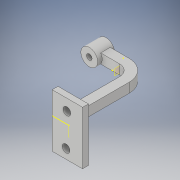
# Autodesk Inventor part: Base
Saved by Autodesk Inventor 2019 (Build 230136000, 136)
## iProperties
Created: 2019-05-09
Part Number: Base
Material: Generic
Document SubType Name: Modeling
Designer: riphipps21
Density: 1 g/cm^3
Appearance: Default
Author: riphipps21
Autodesk Inventor part; units mm, degrees
ref_plane "XZ Plane" through (0, 0, 0) normal (0, 1, 0) x (-1, 0, 0)
ref_plane "XY Plane" through (0, 0, 0) normal (0, 0, 1) x (1, 0, 0)
sketch "Sketch1" plane through (0, 0, 0) normal (0, 0, 1) x (1, 0, 0)
  point P0 (0, 0)
sketch "Sketch2" plane through (0, 0, 0) normal (0, 0, 1) x (1, 0, 0)
  circle A0 centre (-25.9578, 0) radius 5.461
  point P0 (0, 0)
  dimension "d30" = 10.922
  constraints: 1 centre point
  measures "d30" diameter of A0
extrude "Extrusion1" add sketch "Sketch2" along normal blind 12.7 and the other way blind 6.35
sketch "Sketch3" plane through (-25.9578, 0, 12.7) normal (0, 0, 1) x (1, 0, 0)
  point P0 (25.9578, 0)
  point P1 (0.0374, 0.0562)
hole "Hole1" at (-25.9204, 0.0562, 12.7) direction (0, 0, -1) diameter 6.2738 end through all
ref_plane "Work Plane1" through (3.175, 0, 0) normal (1, 0, 0) x (0, 1, 0)
sketch "Sketch4" plane through (3.175, 0, 0) normal (1, 0, 0) x (0, 1, 0)
  line L0 (5.461, -6.35) -> (5.461, 12.7) projected
  line L1 (5.461, 7.62) -> (-5.461, 7.62)
  line L2 (-5.461, 7.62) -> (-5.461, 4.445)
  line L3 (-5.461, 4.445) -> (5.461, 4.445)
  line L4 (5.461, 4.445) -> (5.461, 7.62)
  line L5 (5.461, 12.7) -> (-5.461, 12.7) projected
  line L6 (-5.461, -6.35) -> (-5.461, 12.7) projected
  point P0 (0, 0)
  dimension "d11" = 3.175
  dimension "d12" = 5.08
  constraints: 8 end point, 2 parallel, 1 collinear, 1 horizontal, 1 perpendicular, 1 point on line
  measures "d11" distance between parallel lines of L1 L3
  measures "d12" distance between parallel lines of L1 L5
sketch "Sketch5" plane through (0, 0, 0) normal (0, 1, 0) x (-1, 0, 0)
  line L0 (-3.175, -6.35) -> (-3.175, 12.7) projected
  arc A0 (-15.875, 20.32) -> (-3.175, 7.62) centre (-3.175, 20.32) ccw
  line L1 (-3.175, 20.32) -> (-15.875, 20.32) construction
  line L2 (31.4188, 12.7) -> (20.4968, 12.7) projected
  line L3 (-15.875, 20.32) -> (-15.875, 42.189)
  point P0 (0, 0)
  dimension "d13" = 12.7
  dimension "d14" = 5.08
  dimension "d15" = 0
  constraints: 4 end point, 2 point on circle, 1 centre point, 1 horizontal, 1 point on line, 1 vertical
  measures "d13" radius of A0
  measures "d14" distance from line of L2 A0.end
  measures "d15" distance from line of L1.start L0
sweep "Sweep1" add profiles "Sketch4" path "Sketch5" path curves A0 L3 contours L3 L2 L1 L0
sketch "Sketch8" plane through (3.175, 5.461, 7.62) normal (0, 1, 0) x (1, 0, 0)
  point P0 (-3.175, 7.62)
sketch "Sketch9" plane through (3.175, 5.461, 7.62) normal (0, 1, 0) x (1, 0, 0)
  point P0 (-3.175, 7.62)
sketch "Sketch10" plane through (3.175, 5.461, 7.62) normal (0, 1, 0) x (1, 0, 0)
  point P0 (-3.175, 7.62)
sketch "Sketch11" plane through (3.175, 5.461, 7.62) normal (0, 1, 0) x (1, 0, 0)
  point P0 (-3.175, 7.62)
sketch "Sketch12" plane through (3.175, 5.461, 7.62) normal (0, 1, 0) x (1, 0, 0)
  line L0 (12.7, -34.569) -> (15.875, -34.569) projected
  line L1 (12.7, -34.569) -> (15.875, -34.569)
  line L2 (15.875, -34.569) -> (15.875, -88.8996)
  line L3 (15.875, -88.8996) -> (12.7, -88.8996)
  line L4 (12.7, -88.8996) -> (12.7, -34.569)
  point P0 (-3.175, 7.62)
  constraints: 8 end point, 2 parallel, 1 horizontal, 1 perpendicular
sketch "Sketch13" plane through (3.175, 5.461, 7.62) normal (0, 1, 0) x (1, 0, 0)
  point P0 (-3.175, 7.62)
extrude "Extrusion4" add sketch "Sketch12" against normal blind 10.922
sketch "Sketch14" plane through (3.175, 5.461, 7.62) normal (0, 1, 0) x (1, 0, 0)
  line L0 (15.875, -88.8996) -> (12.7, -88.8996) projected
  line L1 (15.875, -88.8996) -> (31.877, -88.8996)
  line L2 (31.877, -88.8996) -> (31.877, -82.2956)
  line L3 (31.877, -82.2956) -> (15.875, -82.2956)
  line L4 (15.875, -82.2956) -> (15.875, -88.8996)
  point P0 (-3.175, 7.62)
  dimension "d36" = 6.604
  constraints: 8 end point, 2 parallel, 1 horizontal, 1 perpendicular
  measures "d36" distance of L1.end L2.end
extrude "Extrusion5" add sketch "Sketch14" against normal blind 10.922
sketch "Sketch15" plane through (3.175, 5.461, 7.62) normal (0, 1, 0) x (1, 0, 0)
  point P0 (-3.175, 7.62)
sketch "Sketch16" plane through (-25.9578, 0, 12.7) normal (0, 0, 1) x (1, 0, 0)
  point P0 (25.9578, 0)
sketch "Sketch17" plane through (-25.9578, 0, 12.7) normal (0, 0, 1) x (1, 0, 0)
  point P0 (25.9578, 0)
sketch "Sketch18" plane through (3.175, 5.461, 7.62) normal (0, 1, 0) x (1, 0, 0)
  point P0 (-3.175, 7.62)
sketch "Sketch19" plane through (3.175, 0, 0) normal (1, 0, 0) x (0, 1, 0)
  point P0 (0, 0)
sketch "Sketch20" plane through (3.175, 5.1131, 7.62) normal (-1, 0, 0) x (0, 0, 1)
  point P0 (-7.62, -5.1131)
sketch "Sketch21" plane through (3.175, 5.461, 7.62) normal (0, 1, 0) x (1, 0, 0)
  point P0 (-3.175, 7.62)
sketch "Sketch22" plane through (3.175, -5.461, 4.445) normal (-1, 0, 0) x (0, 0, 1)
  point P0 (-4.445, 5.461)
sketch "Sketch23" plane through (3.175, -2.3966, 7.62) normal (-1, 0, 0) x (0, 0, 1)
  point P0 (-7.62, 2.3966)
sketch "Sketch24" plane through (3.175, 5.1131, 7.62) normal (-1, 0, 0) x (0, 0, 1)
  line L0 (-13.97, -10.5741) -> (5.08, -10.5741) projected
  line L1 (-3.175, 0.3479) -> (12.7, 0.3479) projected
  line L2 (-3.1665, -10.5741) -> (0.031, -10.5741)
  line L3 (0.031, -10.5741) -> (0.031, 0.3479)
  line L4 (0.031, 0.3479) -> (-3.1665, 0.3479)
  line L5 (-3.1665, 0.3479) -> (-3.1665, -10.5741)
  point P0 (-7.62, -5.1131)
  point P1 (-3.0587, 0.3479)
  constraints: 8 end point, 2 parallel, 2 point on line, 1 horizontal, 1 perpendicular
extrude "Extrusion6" add sketch "Sketch24" along normal blind 25.4
sketch "Sketch25" plane through (-25.9578, 0, 12.7) normal (0, 0, 1) x (1, 0, 0)
  point P0 (25.9578, 0)
sketch "Sketch26" plane through (-25.9578, 0, 12.7) normal (0, 0, 1) x (1, 0, 0)
  point P0 (25.9578, 0)
sketch "Sketch27" plane through (-25.9578, 0, 12.7) normal (0, 0, 1) x (1, 0, 0)
  point P0 (25.9578, 0)
sketch "Sketch28" plane through (-25.9578, 0, 12.7) normal (0, 0, 1) x (1, 0, 0)
  point P0 (25.9578, 0)
sketch "Sketch29" plane through (-25.9578, 0, 12.7) normal (0, 0, 1) x (1, 0, 0)
  point P0 (25.9578, 0)
sketch "Sketch30" plane through (15.875, 5.461, 96.5196) normal (0, 1, 0) x (1, 0, 0)
  point P0 (-15.875, 96.5196)
thicken "Thicken1" operation add thickness 7.62 both sides no extend neighbours yes toward (1, 0, 0) faces at (19.05, -1.8203, 43.5185) (18.8727, -1.8203, 17.954)
thicken "Thicken2" operation add thickness 7.62 both sides no extend neighbours yes toward (0, 0, -1) faces at (-4.7156, 0, 4.4535)
sketch "Sketch31" plane through (15.875, 5.461, 96.5196) normal (0, 1, 0) x (1, 0, 0)
  line L0 (10.795, 6.604) -> (19.177, 6.604) projected
  line L1 (0, 0) -> (19.177, 0) projected
  line L2 (19.177, 6.604) -> (10.795, 6.604) projected
  line L3 (19.177, 0) -> (19.177, 6.604) projected
  point P0 (-15.875, 96.5196)
ref_plane "Work Plane2" through (35.052, 5.461, 96.5196) normal (1, 0, 0) x (0, 0, -1)
sketch "Sketch32" plane through (35.052, 5.461, 96.5196) normal (1, 0, 0) x (0, 0, -1)
  line L0 (76.1996, 0) -> (0, 0) projected
  line L1 (6.604, 0) -> (6.604, -10.922) projected
  line L2 (0, 0) -> (6.604, 0)
  line L3 (6.604, 0) -> (6.604, -10.922)
  line L4 (6.604, -10.922) -> (0, -10.922)
  line L5 (0, -10.922) -> (0, 0)
  point P0 (96.5196, -5.461)
  constraints: 8 end point, 2 parallel, 1 horizontal, 1 perpendicular
extrude "Extrusion7" add sketch "Sketch32" along normal blind 15.24
thicken "Thicken3" operation add thickness 3.048 both sides no extend neighbours yes toward (-0.4286926, 0.9034504, 0) faces at (-28.2989, 4.9337, 0)
thicken "Thicken4" operation add thickness 1.016 both sides no extend neighbours yes toward (0.6396862, 0.7686362, 0) faces at (-20.5147, 6.5403, 4.667)
sketch "Sketch33" plane through (26.67, -5.461, 89.9156) normal (0, 0, -1) x (-1, 0, 0)
  point P0 (26.67, 5.461)
  point P1 (-18.4473, 5.7167)
hole "Hole2" at (45.1173, 0.2557, 89.9156) direction (0, 0, 1) diameter 8.7884 end through all
sketch "Sketch34" plane through (26.67, -5.461, 89.9156) normal (0, 0, -1) x (-1, 0, 0)
  point P0 (26.67, 5.461)
  point P1 (-6.4339, 5.7203)
hole "Hole3" at (33.1039, 0.2593, 89.9156) direction (0, 0, 1) diameter 8.7884 end through all
sketch "Sketch35" plane through (15.875, 5.461, 96.5196) normal (0, 1, 0) x (1, 0, 0)
  line L0 (10.795, 6.604) -> (34.417, 6.604) projected
  line L1 (0, 0) -> (34.417, 0) projected
  line L2 (0, 76.1996) -> (0, 0) projected
  line L3 (0, 6.604) -> (34.417, 6.604)
  line L4 (34.417, 6.604) -> (34.417, 0)
  line L5 (34.417, 0) -> (0, 0)
  line L6 (0, 0) -> (0, 6.604)
  point P0 (-15.875, 96.5196)
  constraints: 8 end point, 2 parallel, 1 horizontal, 1 perpendicular, 1 point on line
sketch "Sketch36" plane through (15.875, 5.461, 96.5196) normal (0, 1, 0) x (1, 0, 0)
  point P0 (-15.875, 96.5196)
extrude "Extrusion8" add sketch "Sketch35" along normal blind 25.4 and the other way blind 34.925
sketch "Sketch37" plane through (26.67, 5.461, 89.9156) normal (0, 0, -1) x (-1, 0, 0)
  point P0 (26.67, -5.461)
  point P1 (-5.8398, 12.6437)
hole "Hole4" at (32.5098, 18.1047, 89.9156) direction (0, 0, 1) diameter 8.763 end through all
sketch "Sketch38" plane through (26.67, 5.461, 89.9156) normal (0, 0, -1) x (-1, 0, 0)
  point P0 (26.67, -5.461)
  point P1 (-4.9413, -24.2837)
hole "Hole5" at (31.6113, -18.8227, 89.9156) direction (0, 0, 1) diameter 8.763 end through all
body "Solid1"
